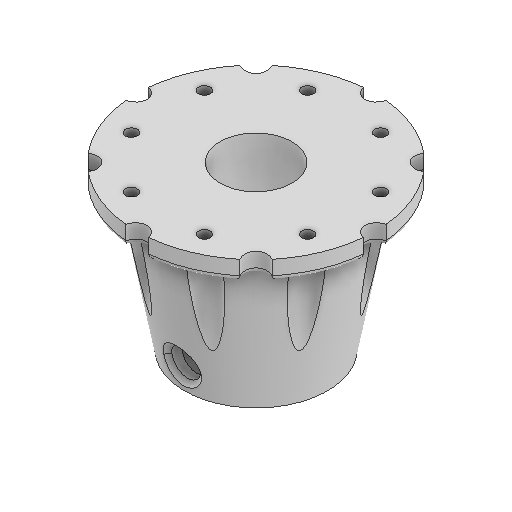
# Autodesk Inventor part: 3DP_ASA_Mast_Mount
Saved by Autodesk Inventor 2026.1 (Build 301233000, 233)
## iProperties
Created: 2025-06-19
Part Number: 3DP_ASA_Mast_Mount
Material: Generic
Document SubType Name: Modeling
Designer: User
Density: 1 g/cm^3
Appearance: Default
Author: User
Autodesk Inventor part; units mm, degrees
ref_plane "YZ Plane" through (0, 0, 0) normal (1, 0, 0) x (0, 1, 0)
sketch "Sketch1" plane through (0, 0, 0) normal (0, 0, 1) x (1, 0, 0)
  line L0 (0, 53.9615) -> (-20, 53.9615)
  line L1 (-20, 53.9615) -> (-50, 2)
  line L2 (-50, 2) -> (-50, 0)
  line L3 (-50, 0) -> (0, 0)
  line L4 (0, 0) -> (0, 53.9615)
  line L5 (0, -10.7923) -> (0, 64.7538) projected
  dimension "d0" = 50
  dimension "d2" = 20
  dimension "d3" = 30
  dimension "d4" = 2
  dimension "d5" = 53.9615
  constraints: 10 end point, 2 perpendicular, 1 horizontal, 1 vertical
  measures "d0" distance between parallel lines of L4 L2
  measures "d2" distance of L0.start L0.end
  measures "d3" angle of L4 L1
  measures "d4" distance of L1.end L2.end
  measures "d5" distance between parallel lines of L3 L0
revolve "Revolution1" add sketch "Sketch1" angle 360 about axis through (0, -10, 0) along (0, 1, 0)
sketch "Sketch2" plane through (0, 53.9615, 0) normal (0, 1, 0) x (1, 0, 0)
  circle A0 centre (0, 0) radius 20 projected
  line L0 (-20, 26.6864) -> (-20, -29.355)
  dimension "d7" = 40
  dimension "d8" = 20
  constraints: 2 end point, 1 vertical
  measures "d7" diameter of A0
  measures "d8" distance from line of point (0, 0) L0
ref_plane "Work Plane1" through (-20, 53.9615, -26.6864) normal (-0.5, -0.8660254, 0) x (0, 0, 1)
sketch "Sketch3" plane through (-20, 53.9615, -26.6864) normal (-0.5, -0.8660254, 0) x (0, 0, 1)
  ellipse E0 centre (26.6864, -43.3013) end of major axis (-23.3136, -43.3013) minor radius 43.3013 projected
  circle A0 centre (26.6864, 0.25) radius 5
  point P0 (26.6864, -44.3013)
  point P1 (26.6864, 0)
  dimension "d11" = 0.25
  dimension "d12" = 10
  constraints: 1 centre point, 1 coincident, 1 vertical alignment, 1 other
  measures "d11" distance of point (26.686, 0) point (26.686, 0.25)
  measures "d12" diameter of A0
extrude "Extrusion1" cut sketch "Sketch3" along normal mid plane 200 contours A0 E0 | E0 A0 picked at (25.0675, -1.4032) picked at (28.4242, 1.4636)
pattern_circular "Circular Pattern1" count 8 over 360 about axis through (0, -10, 0) along (0, 1, 0) of "Extrusion1"
sketch "Sketch4" plane through (0, 53.9615, 0) normal (0, 1, 0) x (0.9238795, 0, 0.3826834)
  point P0 (0, 0)
  point P1 (0, 0)
  constraints: 1 coincident
hole "Hole1" at (0, 53.9615, 0) direction (0, -1, 0) diameter 4 end through all
sketch "Sketch5" plane through (0, 0, 0) normal (0, -1, 0) x (0.9238795, 0, -0.3826834)
  circle A0 centre (0, 0) radius 2 projected
  point P0 (0, 40)
  dimension "d26" = 40
  measures "d26" distance of point (0, 0) point (0, 40)
hole "Hole2" at (15.3073, 0, 36.9552) direction (0, 1, 0) diameter 5 end through all
pattern_circular "Circular Pattern2" count 8 over 360 about axis through (0, -10, 0) along (0, 1, 0) of "Hole2"
sketch "Sketch6" plane through (0, 53.9615, 0) normal (0, 1, 0) x (0.9238795, 0, 0.3826834)
  circle A0 centre (0, 0) radius 2 projected
  circle A1 centre (0, 0) radius 50
  dimension "d37" = 100
  constraints: 1 centre point, 1 coincident
  measures "d37" diameter of A1
extrude "Extrusion2" cut sketch "Sketch6" against normal blind 10
sketch "Sketch7" plane through (0, 0, 0) normal (0, -1, 0) x (0.9238795, 0, -0.3826834)
  circle A0 centre (0, 0) radius 2 projected
  circle A1 centre (0, 0) radius 15.1
  dimension "d40" = 30.2
  constraints: 1 centre point, 1 coincident
  measures "d40" diameter of A1
extrude "Extrusion3" cut sketch "Sketch7" against normal blind 20
sketch "Sketch8" plane through (0, 0, 0) normal (0, -1, 0) x (0.9238795, 0, -0.3826834)
  circle A0 centre (0, 0) radius 15.1 projected
  circle A1 centre (-28.2843, 28.2843) radius 2.5 projected
  circle A2 centre (-40, 0) radius 2.5 projected
  circle A3 centre (-28.2843, -28.2843) radius 2.5 projected
  circle A4 centre (0, -40) radius 2.5 projected
  circle A5 centre (28.2843, -28.2843) radius 2.5 projected
  circle A6 centre (40, 0) radius 2.5 projected
  circle A7 centre (28.2843, 28.2843) radius 2.5 projected
  circle A8 centre (0, 40) radius 2.5 projected
  ellipse E0 centre (-19.6865, -47.5275) end of major axis (-21.896, -52.8615) minor radius 5 (-14.6251, -47.8132) -> (-23.4676, -44.1506) ccw projected
  arc A9 (-14.6251, -47.8132) -> (14.6251, -47.8132) centre (0, 0) ccw projected
  ellipse E1 centre (19.6865, -47.5275) end of major axis (21.896, -52.8615) minor radius 5 (23.4676, -44.1506) -> (14.6251, -47.8132) ccw projected
  arc A10 (23.4676, -44.1506) -> (44.1506, -23.4676) centre (0, 0) ccw projected
  ellipse E2 centre (47.5275, -19.6865) end of major axis (52.8615, -21.896) minor radius 5 (47.8132, -14.6251) -> (44.1506, -23.4676) ccw projected
  arc A11 (47.8132, -14.6251) -> (47.8132, 14.6251) centre (0, 0) ccw projected
  ellipse E3 centre (47.5275, 19.6865) end of major axis (52.8615, 21.896) minor radius 5 (44.1506, 23.4676) -> (47.8132, 14.6251) ccw projected
  arc A12 (44.1506, 23.4676) -> (23.4676, 44.1506) centre (0, 0) ccw projected
  ellipse E4 centre (19.6865, 47.5275) end of major axis (21.896, 52.8615) minor radius 5 (14.6251, 47.8132) -> (23.4676, 44.1506) ccw projected
  arc A13 (14.6251, 47.8132) -> (-14.6251, 47.8132) centre (0, 0) ccw projected
  ellipse E5 centre (-19.6865, 47.5275) end of major axis (-21.896, 52.8615) minor radius 5 (-23.4676, 44.1506) -> (-14.6251, 47.8132) ccw projected
  arc A14 (-23.4676, 44.1506) -> (-44.1506, 23.4676) centre (0, 0) ccw projected
  ellipse E6 centre (-47.5275, 19.6865) end of major axis (-52.8615, 21.896) minor radius 5 (-47.8132, 14.6251) -> (-44.1506, 23.4676) ccw projected
  arc A15 (-47.8132, 14.6251) -> (-47.8132, -14.6251) centre (0, 0) ccw projected
  ellipse E7 centre (-47.5275, -19.6865) end of major axis (-52.8615, -21.896) minor radius 5 (-44.1506, -23.4676) -> (-47.8132, -14.6251) ccw projected
  arc A16 (-44.1506, -23.4676) -> (-23.4676, -44.1506) centre (0, 0) ccw projected
  circle A17 centre (0, 0) radius 2 projected
  circle A18 centre (0, 0) radius 60
  dimension "d43" = 120
  constraints: 1 centre point, 1 coincident, 8 other
  measures "d43" diameter of A18
extrude "Extrusion4" cut sketch "Sketch8" against normal through all contours A0 | E0 A16 E7 A15 E6 A14 E5 A13 E4 A12 E3 A11 E2 A10 E1 A9 | A18
extrude "Extrusion5" add sketch "Sketch8" along normal blind 8 contours E0 A16 E7 A15 E6 A14 E5 A13 E4 A12 E3 A11 E2 A10 E1 A9
sketch "Sketch9" plane through (0, -8, 0) normal (0, -1, 0) x (0.9238795, 0, -0.3826834)
  circle A0 centre (0, 0) radius 30
  circle A1 centre (0, 0) radius 15.1 projected
  dimension "d48" = 60
  constraints: 1 centre point, 1 coincident
  measures "d48" diameter of A0
extrude "Extrusion6" add sketch "Sketch9" along normal blind 60
chamfer "Chamfer1" distance 11 distance2 60 1 edges at (-27.7164, -8, 11.4805)
sketch "Sketch10" plane through (0, -8, 0) normal (0, -1, 0) x (0.9238795, 0, -0.3826834)
  arc A0 (-40.9344, -2.3188) -> (-30.5846, -27.3053) centre (0, 0) ccw projected
  arc A1 (-40.9344, 2.3188) -> (-40.9344, -2.3188) centre (-40, 0) ccw projected
  arc A2 (-30.5846, 27.3053) -> (-40.9344, 2.3188) centre (0, 0) ccw projected
  arc A3 (-27.3053, 30.5846) -> (-30.5846, 27.3053) centre (-28.2843, 28.2843) ccw projected
  arc A4 (-2.3188, 40.9344) -> (-27.3053, 30.5846) centre (0, 0) ccw projected
  arc A5 (2.3188, 40.9344) -> (-2.3188, 40.9344) centre (0, 40) ccw projected
  arc A6 (27.3053, 30.5846) -> (2.3188, 40.9344) centre (0, 0) ccw projected
  arc A7 (30.5846, 27.3053) -> (27.3053, 30.5846) centre (28.2843, 28.2843) ccw projected
  arc A8 (40.9344, 2.3188) -> (30.5846, 27.3053) centre (0, 0) ccw projected
  arc A9 (40.9344, -2.3188) -> (40.9344, 2.3188) centre (40, 0) ccw projected
  arc A10 (30.5846, -27.3053) -> (40.9344, -2.3188) centre (0, 0) ccw projected
  arc A11 (27.3053, -30.5846) -> (30.5846, -27.3053) centre (28.2843, -28.2843) ccw projected
  arc A12 (2.3188, -40.9344) -> (27.3053, -30.5846) centre (0, 0) ccw projected
  arc A13 (-2.3188, -40.9344) -> (2.3188, -40.9344) centre (0, -40) ccw projected
  arc A14 (-27.3053, -30.5846) -> (-2.3188, -40.9344) centre (0, 0) ccw projected
  arc A15 (-30.5846, -27.3053) -> (-27.3053, -30.5846) centre (-28.2843, -28.2843) ccw projected
  ellipse E0 centre (47.5275, -19.6865) end of major axis (42.1935, -17.4771) minor radius 5 (47.8132, -14.6251) -> (44.1506, -23.4676) ccw projected
  arc A16 (47.8132, -14.6251) -> (47.8132, 14.6251) centre (0, 0) ccw projected
  ellipse E1 centre (47.5275, 19.6865) end of major axis (42.1935, 17.4771) minor radius 5 (44.1506, 23.4676) -> (47.8132, 14.6251) ccw projected
  arc A17 (44.1506, 23.4676) -> (23.4676, 44.1506) centre (0, 0) ccw projected
  ellipse E2 centre (19.6865, 47.5275) end of major axis (17.4771, 42.1935) minor radius 5 (14.6251, 47.8132) -> (23.4676, 44.1506) ccw projected
  arc A18 (14.6251, 47.8132) -> (-14.6251, 47.8132) centre (0, 0) ccw projected
  ellipse E3 centre (-19.6865, 47.5275) end of major axis (-17.4771, 42.1935) minor radius 5 (-23.4676, 44.1506) -> (-14.6251, 47.8132) ccw projected
  arc A19 (-23.4676, 44.1506) -> (-44.1506, 23.4676) centre (0, 0) ccw projected
  ellipse E4 centre (-47.5275, 19.6865) end of major axis (-42.1935, 17.4771) minor radius 5 (-47.8132, 14.6251) -> (-44.1506, 23.4676) ccw projected
  arc A20 (-47.8132, 14.6251) -> (-47.8132, -14.6251) centre (0, 0) ccw projected
  ellipse E5 centre (-47.5275, -19.6865) end of major axis (-42.1935, -17.4771) minor radius 5 (-44.1506, -23.4676) -> (-47.8132, -14.6251) ccw projected
  arc A21 (-44.1506, -23.4676) -> (-23.4676, -44.1506) centre (0, 0) ccw projected
  ellipse E6 centre (-19.6865, -47.5275) end of major axis (-17.4771, -42.1935) minor radius 5 (-14.6251, -47.8132) -> (-23.4676, -44.1506) ccw projected
  arc A22 (-14.6251, -47.8132) -> (14.6251, -47.8132) centre (0, 0) ccw projected
  ellipse E7 centre (19.6865, -47.5275) end of major axis (17.4771, -42.1935) minor radius 5 (23.4676, -44.1506) -> (14.6251, -47.8132) ccw projected
  arc A23 (23.4676, -44.1506) -> (44.1506, -23.4676) centre (0, 0) ccw projected
  circle A24 centre (0, 40) radius 6
  circle A25 centre (-28.2843, 28.2843) radius 6
  circle A26 centre (-40, 0) radius 6
  circle A27 centre (-28.2843, -28.2843) radius 6
  circle A28 centre (0, -40) radius 6
  circle A29 centre (28.2843, -28.2843) radius 6
  circle A30 centre (40, 0) radius 6
  circle A31 centre (28.2843, 28.2843) radius 2.5 projected
  circle A32 centre (28.2843, 28.2843) radius 6
  dimension "d54" = 12
  dimension "d55" = 12
  dimension "d56" = 12
  dimension "d57" = 12
  dimension "d58" = 12
  dimension "d59" = 12
  dimension "d60" = 12
  dimension "d61" = 12
  constraints: 8 centre point, 8 coincident, 8 other
  measures "d54" diameter of A24
  measures "d55" diameter of A25
  measures "d56" diameter of A26
  measures "d57" diameter of A27
  measures "d58" diameter of A28
  measures "d59" diameter of A29
  measures "d60" diameter of A30
  measures "d61" diameter of A32
extrude "Extrusion7" cut sketch "Sketch10" along normal through all contours A1 A2 A26 A0 | A0 A26 A2 A1 | A27 A14 A15 A0 | A0 A15 A14 A27 | A25 A4 A3 A2 | A2 A3 A4 A25 | A28 A12 A13 A14 | A14 A13 A12 A28 | A24 A6 A5 A4 | A4 A5 A6 A24 | A29 A10 A11 A12 | A12 A11 A10 A29 | A32 A8 A7 A6 | A6 A31 A8 A32 | A30 A8 A9 A10 | A10 A9 A8 A30
ref_plane "Work Plane2" through (0, 0, 25) normal (0, 0, 1) x (1, 0, 0)
sketch "Sketch11" plane through (0, 0, 25) normal (0, 0, 1) x (1, 0, 0)
  circle A0 centre (0, -58) radius 2.5
  line L0 (15.1, -68) -> (-15.1, -68) projected
  circle A1 centre (0, -58) radius 6
  point P0 (0, 0)
  dimension "d65" = 5
  dimension "d66" = 10
  dimension "d69" = 12
  constraints: 2 centre point, 1 coincident
  measures "d65" diameter of A0
  measures "d66" distance from line of L0 A0.centre
  measures "d69" diameter of A1
extrude "Extrusion8" cut sketch "Sketch11" along normal through all both and the other way through all contours A0
extrude "Extrusion9" cut sketch "Sketch11" along normal blind 10
chamfer "Chamfer2" distance 2 angle 45 1 edges at (-5.9982, -57.8523, 31.2907)
mirror "Mirror1" about plane through (0, 0, 0) normal (0, 0, 1) of "Extrusion9", "Chamfer2"
fillet "Fillet1" radius 2 16 edges at (-19.1342, -8, -46.194) (-32.2935, -8, -32.2935) (-46.194, -8, -19.1342) (-45.6699, -8, 0) (-46.194, -8, 19.1342) (-32.2935, -8, 32.2935) (-19.1342, -8, 46.194) (0, -8, 45.6699) (19.1342, -8, 46.194) (32.2935, -8, 32.2935) (46.194, -8, 19.1342) (45.6699, -8, 0) (46.194, -8, -19.1342) (32.2935, -8, -32.2935) (19.1342, -8, -46.194) (0, -8, -45.6699)
equation "\"d8\" = 0.5 * d7"
body "Solid1"
